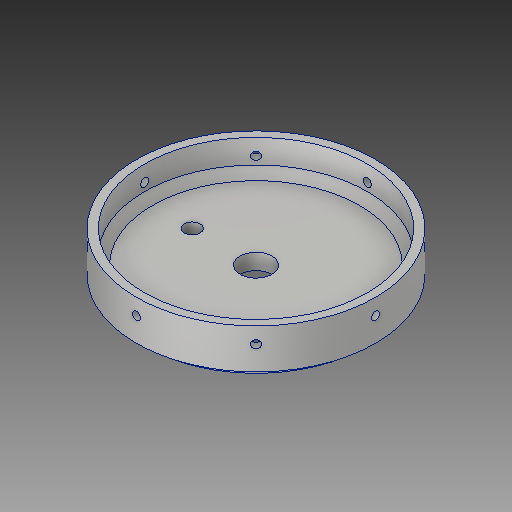
# Autodesk Inventor part: motor_bulkhead
Saved by Autodesk Inventor 2017 SP1 (Build 210196100, 196)
## iProperties
Created: 2016-10-29
Part Number: motor_bulkhead
Material: Aluminum 6061
Document SubType Name: Modeling
Designer: cflannery
Density: 2.7 g/cm^3
Appearance: Aluminum - Flat
Mass: 1157.84 g
Surface Area: 923.175 cm^2
Volume: 428.829 cm^3
Author: cflannery
Autodesk Inventor part; units mm, degrees
ref_plane "YZ Plane" through (0, 0, 0) normal (1, 0, 0) x (0, 1, 0)
ref_plane "XZ Plane" through (0, 0, 0) normal (0, 1, 0) x (-1, 0, 0)
sketch "Sketch1" plane through (0, 0, 0) normal (0, 1, 0) x (-1, 0, 0)
  circle A0 centre (0, 0) radius 87.63
  dimension "d0" = 175.26
  constraints: 1 centre point, 1 coincident
  measures "d0" diameter of A0
extrude "Extrusion1" add sketch "Sketch1" along normal blind 6.35
sketch "Sketch2" plane through (0, 6.35, 0) normal (0, 1, 0) x (1, 0, 0)
  circle A0 centre (0, 0) radius 95.25
  dimension "d3" = 190.5
  constraints: 1 centre point, 1 coincident
  measures "d3" diameter of A0
extrude "Extrusion2" add sketch "Sketch2" along normal blind 6.35
sketch "Sketch3" plane through (0, 12.7, 0) normal (0, 1, 0) x (1, 0, 0)
  circle A0 centre (0, 0) radius 88.9
  circle A1 centre (0, 0) radius 95.25
  dimension "d6" = 190.5
  dimension "d7" = 177.8
  constraints: 2 centre point, 2 coincident
  measures "d6" diameter of A1
  measures "d7" diameter of A0
extrude "Extrusion3" add sketch "Sketch3" along normal blind 25.4
ref_plane "Work Plane1" through (0, 6.35, 95.25) normal (0, 0, 1) x (1, 0, 0)
sketch "Sketch4" plane through (0, 6.35, 95.25) normal (0, 0, 1) x (1, 0, 0)
  line L0 (-95.25, 0) -> (95.25, 0) projected
  point P0 (0, -6.35)
  point P1 (0, 19.05)
  dimension "d10" = 19.05
  measures "d10" distance from line of L0 point (0, 19.05)
hole "Hole1" at (0, 25.4, 95.25) direction (0, 0, -1) diameter 6.35 depth 25.4 tip angle 118
pattern_circular "Circular Pattern1" count 8 over 360 about axis through (0, 6.35, 0) along (0, 1, 0) of "Hole1"
sketch "Sketch5" plane through (0, 12.7, 0) normal (0, 1, 0) x (1, 0, 0)
  circle A0 centre (0, 0) radius 12.7
  circle A1 centre (-50.8, 0) radius 6.35
  dimension "d21" = 12.7
  dimension "d22" = 25.4
  dimension "d23" = 50.8
  constraints: 2 centre point, 1 coincident, 1 horizontal alignment
  measures "d21" diameter of A1
  measures "d22" diameter of A0
  measures "d23" distance of point (0, 0) A1.centre
extrude "Extrusion4" cut sketch "Sketch5" against normal blind 12.7
chamfer "Chamfer1" distance 6.35 angle 45 1 edges at (-88.9, 12.7, 0)
body "Solid1"
